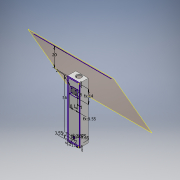
# Autodesk Inventor part: QC25BTFication_2
Saved by Autodesk Inventor 2018 (Build 220112000, 112)
## iProperties
Created: 2021-09-19
Part Number: QC25BTFication_2
Material: Generic
Document SubType Name: Modeling
Designer: dangl
Density: 1 g/cm^3
Appearance: Default
Author: dangl
Autodesk Inventor part; units mm, degrees
ref_plane "YZ Plane" through (0, 0, 0) normal (1, 0, 0) x (0, 1, 0)
ref_plane "XZ Plane" through (0, 0, 0) normal (0, 1, 0) x (-1, 0, 0)
ref_plane "XY Plane" through (0, 0, 0) normal (0, 0, 1) x (1, 0, 0)
sketch "Sketch3" plane through (0, 0, 0) normal (0, 1, 0) x (-1, 0, 0)
  line L0 (0, 0) -> (11, 0)
  line L1 (11, 0) -> (11, -56)
  line L2 (11, -56) -> (0, -56)
  line L3 (0, -56) -> (0, 0)
  line L4 (12, 1) -> (-1, 1)
  line L5 (-1, 1) -> (-1, -57)
  line L6 (-1, -57) -> (12, -57)
  line L7 (12, -57) -> (12, 1)
  line L8 (7.55, -6.2) -> (3.45, -6.2)
  line L9 (1.45, -8.2) -> (1.45, -12)
  line L10 (3.45, -14) -> (7.55, -14)
  line L11 (9.55, -12) -> (9.55, -8.2)
  arc A0 (9.55, -8.2) -> (7.55, -6.2) centre (7.55, -8.2) ccw
  arc A1 (7.55, -14) -> (9.55, -12) centre (7.55, -12) ccw
  arc A2 (1.45, -12) -> (3.45, -14) centre (3.45, -12) ccw
  arc A3 (3.45, -6.2) -> (1.45, -8.2) centre (3.45, -8.2) ccw
  circle A4 centre (5.5, -51) radius 1
  point P0 (1.45, -14)
  point P1 (1.45, -6.2)
  point P2 (9.55, -14)
  dimension "d2" = 11
  dimension "d3" = 56
  dimension "d4" = 1
  dimension "d5" = 1
  dimension "d6" = 1
  dimension "d7" = 1
  dimension "d8" = 8.1
  dimension "d9" = 7.8
  dimension "d10" = 14
  dimension "d11" = 9.55
  dimension "d12" = 2
  dimension "d30" = 2
  dimension "d31" = 5
  dimension "d32" = 5.5
  constraints: 24 end point, 8 point on circle, 8 tangent, 6 parallel, 6 point on line, 5 centre point, 3 equal radius, 3 horizontal, 3 perpendicular
  measures "d2" distance of L1.end L2.end
  measures "d3" distance of L0.end L1.end
  measures "d4" distance between parallel lines of L1 L7
  measures "d5" distance between parallel lines of L2 L6
  measures "d6" distance between parallel lines of L0 L4
  measures "d7" distance between parallel lines of L5 L3
  measures "d8" distance of point (1.45, -14) point (9.55, -14)
  measures "d9" distance of point (1.45, -6.2) point (1.45, -14)
  measures "d10" distance between parallel lines of L0 L10
  measures "d11" distance between parallel lines of L3 L11
  measures "d12" radius of A0
  measures "d30" diameter of A4
  measures "d31" distance from line of L2 A4.centre
  measures "d32" distance from line of L3 A4.centre
extrude "Extrusion1" add sketch "Sketch3" along normal blind 1.4 contours L0 L1 L2 L3
extrude "Extrusion3" add sketch "Sketch3" along normal blind 8.6 contours L7 L6 L5 L4
sketch "Sketch4" plane through (-12, 0, 1) normal (0, 0, 1) x (1, 0, 0)
  circle A0 centre (6.5, 5.4) radius 2.65
  line L0 (0, 0) -> (0, 8.6) projected
  line L1 (0, 0) -> (13, 0) projected
  point P0 (12, 0)
  dimension "d19" = 6.5
  dimension "d20" = 5.3
  dimension "d21" = 5.4
  constraints: 1 centre point
  measures "d19" distance from line of L0 A0.centre
  measures "d20" diameter of A0
  measures "d21" distance from line of L1 A0.centre
extrude "Extrusion4" cut sketch "Sketch4" against normal blind 8.6
sketch "Sketch5" plane through (1, 0, -57) normal (0, 0, -1) x (-1, 0, 0)
  line L0 (2.675, 6.25) -> (10.325, 6.25)
  line L1 (10.325, 6.25) -> (10.325, 3.55)
  line L2 (10.325, 3.55) -> (2.675, 3.55)
  line L3 (2.675, 3.55) -> (2.675, 6.25)
  line L4 (0, 0) -> (13, 0) projected
  line L5 (13, 0) -> (13, 8.6) projected
  point P0 (1, 0)
  dimension "d24" = 7.65
  dimension "d25" = 2.7
  dimension "d26" = 3.55
  dimension "d27" = 2.675
  constraints: 8 end point, 2 parallel, 1 horizontal, 1 perpendicular
  measures "d24" distance of L0.start L0.end
  measures "d25" distance of L0.end L1.end
  measures "d26" distance between parallel lines of L4 L2
  measures "d27" distance between parallel lines of L5 L1
extrude "Extrusion5" cut sketch "Sketch5" against normal blind 8.6
sketch "Sketch6" plane through (0, 0, 0) normal (0, 1, 0) x (-1, 0, 0)
  line L0 (46.885, 21) -> (-33.7151, 21)
  line L1 (12, 1) -> (-1, 1) projected
  point P0 (0, 0)
  dimension "d33" = 20
  constraints: 2 end point, 1 horizontal
  measures "d33" distance between parallel lines of L1 L0
ref_plane "Work Plane1" through (-46.885, 0, 21) normal (0, -0.8660254, -0.5) x (1, 0, 0)
equation "\"d11\" = 0.5 * d2 + 0.5 * d8"
equation "\"d32\" = 0.5 * d2"
equation "\"d19\" = 0.5 * d2 + d4"
body "Solid1"
